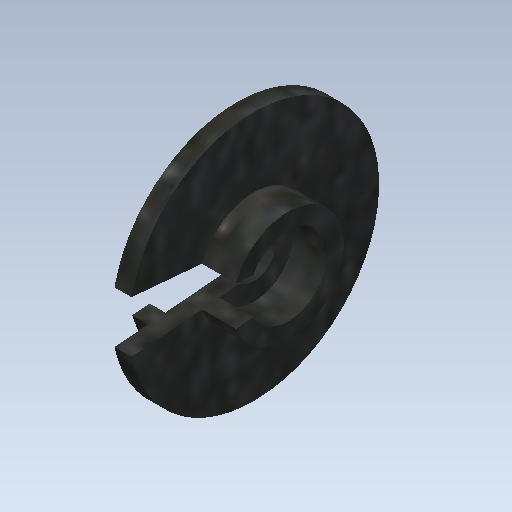
# Autodesk Inventor part: 500-105
Saved by Autodesk Inventor 2020 (Build 240168000, 168)
## iProperties
Created: 2015-04-18
Part Number: 500-105
Material: Steel
Document SubType Name: Modeling
Designer: Station9
Density: 7.85 g/cm^3
Appearance: Plate
Mass: 3.52113 g
Surface Area: 8.08268 cm^2
Volume: 0.448551 cm^3
Author: Station9
Autodesk Inventor part; units mm, degrees
ref_plane "YZ Plane" through (0, 0, 0) normal (1, 0, 0) x (0, 1, 0)
ref_plane "XZ Plane" through (0, 0, 0) normal (0, 1, 0) x (-1, 0, 0)
ref_plane "XY Plane" through (0, 0, 0) normal (0, 0, 1) x (1, 0, 0)
sketch "Sketch1" plane through (0, 0, 0) normal (0, 1, 0) x (-1, 0, 0)
  line L0 (5.1, 7) -> (3.9, 7)
  line L1 (3.9, 7) -> (3.9, 9.55)
  line L2 (3.9, 9.55) -> (2.6, 9.55)
  line L3 (2.6, 9.55) -> (2.6, 4.25)
  line L4 (2.6, 4.25) -> (0, 4.25)
  line L5 (0, 4.25) -> (0, 3)
  line L6 (0, 3) -> (2.6, 3)
  line L7 (2.6, 3) -> (2.6, 1.65)
  line L8 (2.6, 1.65) -> (3.9, 1.65)
  line L9 (3.9, 1.65) -> (3.9, 5.7)
  line L10 (3.9, 5.7) -> (5.1, 5.7)
  line L11 (5.1, 5.7) -> (5.1, 7)
  line L12 (0, -1.91) -> (0, 11.46) projected
  line L13 (6.12, 0) -> (-1.02, 0) projected
  point P0 (0, 0)
  dimension "d0" = 5.1
  dimension "d1" = 4.25
  dimension "d2" = 3
  dimension "d3" = 1.65
  dimension "d4" = 1.3
  dimension "d5" = 2.5
  dimension "d6" = 0
  dimension "d7" = 9.55
  dimension "d8" = 7
  dimension "d9" = 5.7
  constraints: 24 end point, 6 perpendicular, 3 parallel, 2 horizontal, 2 vertical alignment, 1 vertical
  measures "d0" distance between parallel lines of L5 L11
  measures "d1" distance from line of point (0, 0) L4
  measures "d2" distance from line of point (0, 0) L6
  measures "d3" distance from line of point (0, 0) L8
  measures "d4" distance of L1.end L2.end
  measures "d5" distance between parallel lines of L3 L11
  measures "d6" distance from line of point (0, 0) L5
  measures "d7" distance from line of point (0, 0) L2
  measures "d8" distance from line of point (0, 0) L0
  measures "d9" distance from line of point (0, 0) L10
revolve "Revolution2" add sketch "Sketch1" angle 360 about axis through (-10, 0, 0) along (1, 0, 0)
sketch "Sketch2" plane through (-5.1, 0, 0) normal (-1, 0, 0) x (0, 0, 1)
  circle A0 centre (0, 0) radius 7 projected
  circle A1 centre (0, 0) radius 1.65 projected
  line L0 (1.077, -1.25) -> (11.1995, -2.1356)
  line L1 (1.077, -1.25) -> (11.2382, -1.25) construction
  line L2 (1.077, 1.25) -> (12.5248, 2.2516)
  line L3 (1.077, 1.25) -> (12.5685, 1.25) construction
  line L4 (11.1995, -2.1356) -> (12.5248, 2.2516)
  dimension "d12" = 5
  dimension "d13" = 5
  dimension "d14" = 2.5
  dimension "d15" = 1.25
  constraints: 10 end point, 2 equal length, 2 horizontal, 2 point on circle
  measures "d12" angle of L0 L1
  measures "d13" angle of L3 L2
  measures "d14" distance of L2.start L0.start
  measures "d15" vertical distance of A0.centre L2.start
extrude "Extrusion1" cut sketch "Sketch2" against normal through all contours A0 L0 A1 L2 | A0 L2 L4 L0 picked at (5.1628, 0.7044)
equation "\"d15\" = 0.5 * d14"
body "Solid2"
